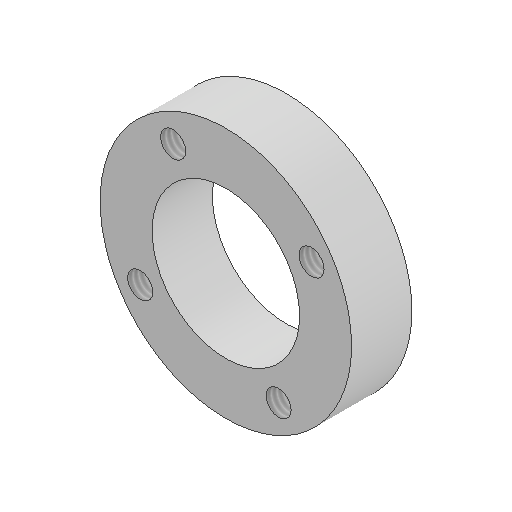
# Autodesk Inventor part: Part16
Saved by Autodesk Inventor 2024 (Build 280153000, 153)
## iProperties
Created: 2023-04-05
Part Number: Part16
Material: Generic
Document SubType Name: Modeling
Designer: ralph
Density: 1 g/cm^3
Appearance: Default
Author: ralph
Autodesk Inventor part; units mm, degrees
ref_plane "YZ Plane" through (0, 0, 0) normal (1, 0, 0) x (0, 1, 0)
ref_plane "XZ Plane" through (0, 0, 0) normal (0, 1, 0) x (-1, 0, 0)
ref_plane "XY Plane" through (0, 0, 0) normal (0, 0, 1) x (1, 0, 0)
sketch "Sketch1" plane through (0, 0, 0) normal (0, 0, 1) x (1, 0, 0)
  circle A0 centre (0, -5) radius 23.8125
  ellipse E0 centre (-25.0666, -29.0096) end of major axis (-17.3967, -26.4903) minor radius 5.8789 (-26.9076, -23.4263) -> (-26.9076, -23.4263) ccw projected
  line L0 (-26.9076, -23.4263) -> (-27.832, -23.7377) projected
  line L1 (-29.2659, -21.4083) -> (-28.5247, -20.677) projected
  ellipse E1 centre (-32.7272, -16.5643) end of major axis (-27.023, -10.8513) minor radius 5.8792 (-28.5715, -20.7232) -> (-28.5252, -20.6765) ccw projected
  ellipse E2 centre (-32.3466, -17.5895) end of major axis (-24.2964, -18.1971) minor radius 5.879 (-31.9108, -11.7266) -> (-31.9108, -11.7266) ccw projected
  line L2 (-31.9108, -11.7266) -> (-32.884, -11.6605) projected
  line L3 (-33.3173, -8.9597) -> (-32.3527, -8.5677) projected
  ellipse E3 centre (-34.6613, -3.1603) end of major axis (-27.2053, -0.0652) minor radius 5.8788 (-32.4136, -8.5925) -> (-32.353, -8.5671) ccw projected
  ellipse E4 centre (-34.7021, -4.2527) end of major axis (-41.907, -0.6107) minor radius 5.8791 (-32.0559, 0.9971) -> (-32.0559, 0.9971) ccw projected
  line L4 (-32.0559, 0.9971) -> (-32.9298, 1.4307) projected
  line L5 (-32.2965, 4.0917) -> (-31.2553, 4.0847) projected
  ellipse E5 centre (-31.3188, 9.9638) end of major axis (-23.246, 9.97) minor radius 5.8786 (-31.321, 4.0851) -> (-31.2553, 4.0853) ccw projected
  ellipse E6 centre (-31.7749, 8.9701) end of major axis (-37.0377, 15.0923) minor radius 5.8794 (-27.3208, 12.8079) -> (-27.3208, 12.8079) ccw projected
  line L6 (-27.3208, 12.8079) -> (-27.9622, 13.5428) projected
  line L7 (-26.3588, 15.759) -> (-25.3996, 15.3541) projected
  ellipse E7 centre (-23.2082, 20.8106) end of major axis (-30.6693, 23.8943) minor radius 5.8793 (-25.4601, 15.3796) -> (-25.3993, 15.3547) ccw projected
  ellipse E8 centre (-24.0096, 20.0665) end of major axis (-26.5289, 27.7364) minor radius 5.8789 (-18.4263, 21.9076) -> (-18.4263, 21.9076) ccw projected
  line L8 (-18.4263, 21.9076) -> (-18.7377, 22.832) projected
  line L9 (-16.4083, 24.2659) -> (-15.677, 23.5247) projected
  ellipse E9 centre (-11.5646, 27.7269) end of major axis (-17.2775, 33.4309) minor radius 5.8788 (-15.7232, 23.5715) -> (-15.6765, 23.5252) ccw projected
  ellipse E10 centre (-12.5894, 27.3465) end of major axis (-11.9818, 35.3967) minor radius 5.8789 (-6.7266, 26.9108) -> (-6.7266, 26.9108) ccw projected
  line L10 (-6.7266, 26.9108) -> (-6.6605, 27.884) projected
  line L11 (-3.9597, 28.3173) -> (-3.5677, 27.3527) projected
  ellipse E11 centre (1.8398, 29.6613) end of major axis (-1.2553, 37.1175) minor radius 5.879 (-3.5925, 27.4136) -> (-3.5671, 27.353) ccw projected
  ellipse E12 centre (0.7479, 29.7018) end of major axis (4.3898, 36.9062) minor radius 5.8783 (5.9971, 27.0559) -> (5.9971, 27.0559) ccw projected
  line L12 (5.9971, 27.0559) -> (6.4307, 27.9298) projected
  line L13 (9.0917, 27.2965) -> (9.0847, 26.2553) projected
  ellipse E13 centre (14.9639, 26.3188) end of major axis (14.9577, 34.3917) minor radius 5.8788 (9.0851, 26.321) -> (9.0853, 26.2553) ccw projected
  ellipse E14 centre (13.9703, 26.7747) end of major axis (20.0923, 32.0374) minor radius 5.8792 (17.8079, 22.3208) -> (17.8079, 22.3208) ccw projected
  line L14 (17.8079, 22.3208) -> (18.5428, 22.9622) projected
  line L15 (20.759, 21.3588) -> (20.3541, 20.3996) projected
  ellipse E15 centre (25.8103, 18.2083) end of major axis (28.8939, 25.6692) minor radius 5.879 (20.3796, 20.4601) -> (20.3547, 20.3993) ccw projected
  ellipse E16 centre (25.0664, 19.0099) end of major axis (32.7365, 21.5293) minor radius 5.8793 (26.9076, 13.4263) -> (26.9076, 13.4263) ccw projected
  line L16 (26.9076, 13.4263) -> (27.832, 13.7377) projected
  line L17 (29.2659, 11.4083) -> (28.5247, 10.677) projected
  ellipse E17 centre (32.7273, 6.5642) end of major axis (38.4316, 12.2773) minor radius 5.8794 (28.5715, 10.7232) -> (28.5252, 10.6765) ccw projected
  ellipse E18 centre (32.3466, 7.5897) end of major axis (40.3969, 6.9821) minor radius 5.8792 (31.9108, 1.7266) -> (31.9108, 1.7266) ccw projected
  line L18 (31.9108, 1.7266) -> (32.884, 1.6605) projected
  line L19 (33.3173, -1.0403) -> (32.3527, -1.4323) projected
  ellipse E19 centre (34.6614, -6.8401) end of major axis (42.1177, -3.7449) minor radius 5.8793 (32.4136, -1.4075) -> (32.353, -1.4329) ccw projected
  ellipse E20 centre (34.702, -5.7476) end of major axis (27.4973, -2.1056) minor radius 5.8787 (32.0559, -10.9971) -> (32.0559, -10.9971) ccw projected
  line L20 (32.0559, -10.9971) -> (32.9298, -11.4307) projected
  line L21 (32.2965, -14.0917) -> (31.2553, -14.0847) projected
  ellipse E21 centre (31.3188, -19.9647) end of major axis (39.3922, -19.9584) minor radius 5.8795 (31.321, -14.0851) -> (31.2553, -14.0853) ccw projected
  ellipse E22 centre (31.7746, -18.9703) end of major axis (26.5119, -12.8483) minor radius 5.8791 (27.3208, -22.8079) -> (27.3208, -22.8079) ccw projected
  line L22 (27.3208, -22.8079) -> (27.9622, -23.5428) projected
  line L23 (26.3588, -25.759) -> (25.3996, -25.3541) projected
  ellipse E23 centre (23.2082, -30.8104) end of major axis (15.7472, -27.7267) minor radius 5.8792 (25.4601, -25.3796) -> (25.3993, -25.3547) ccw projected
  ellipse E24 centre (24.0098, -30.0665) end of major axis (21.4905, -22.3965) minor radius 5.8792 (18.4263, -31.9076) -> (18.4263, -31.9076) ccw projected
  line L24 (18.4263, -31.9076) -> (18.7377, -32.832) projected
  line L25 (16.4083, -34.2659) -> (15.677, -33.5247) projected
  ellipse E25 centre (11.5644, -37.7271) end of major axis (5.8515, -32.0229) minor radius 5.8791 (15.7232, -33.5715) -> (15.6765, -33.5252) ccw projected
  ellipse E26 centre (12.5894, -37.3465) end of major axis (13.197, -29.2964) minor radius 5.879 (6.7266, -36.9108) -> (6.7266, -36.9108) ccw projected
  line L26 (6.7266, -36.9108) -> (6.6605, -37.884) projected
  line L27 (3.9597, -38.3173) -> (3.5677, -37.3527) projected
  ellipse E27 centre (-1.84, -39.6614) end of major axis (-4.9353, -32.2052) minor radius 5.8792 (3.5925, -37.4136) -> (3.5671, -37.353) ccw projected
  ellipse E28 centre (-0.7476, -39.702) end of major axis (2.8944, -32.4973) minor radius 5.8788 (-5.9971, -37.0559) -> (-5.9971, -37.0559) ccw projected
  line L28 (-5.9971, -37.0559) -> (-6.4307, -37.9298) projected
  line L29 (-9.0917, -37.2965) -> (-9.0847, -36.2553) projected
  ellipse E29 centre (-14.9646, -36.3188) end of major axis (-14.9708, -28.2455) minor radius 5.8794 (-9.0851, -36.321) -> (-9.0853, -36.2553) ccw projected
  ellipse E30 centre (-13.9704, -36.7745) end of major axis (-7.8485, -31.5119) minor radius 5.8789 (-17.8079, -32.3208) -> (-17.8079, -32.3208) ccw projected
  line L30 (-17.8079, -32.3208) -> (-18.5428, -32.9622) projected
  line L31 (-20.759, -31.3588) -> (-20.3541, -30.3996) projected
  ellipse E31 centre (-25.8105, -28.2082) end of major axis (-22.7268, -20.7472) minor radius 5.8792 (-20.3796, -30.4601) -> (-20.3547, -30.3993) ccw projected
  arc A1 (-20.3547, -30.3993) -> (-19.6444, -27.7629) centre (-30.6222, -26.2195) ccw projected
  arc A2 (-19.6444, -27.7629) -> (-24.163, -22.8941) centre (-23.8575, -27.1418) ccw projected
  arc A3 (-24.163, -22.8941) -> (-26.8451, -23.406) centre (-23.4417, -33.9564) ccw projected
  arc A4 (-28.5252, -20.6765) -> (-26.86, -18.5126) centre (-36.4116, -12.8856) ccw projected
  arc A5 (-26.86, -18.5126) -> (-29.1715, -12.2852) centre (-30.5148, -16.3265) ccw projected
  arc A6 (-29.1715, -12.2852) -> (-31.8453, -11.7317) centre (-32.7384, -22.7815) ccw projected
  arc A7 (-32.353, -8.5671) -> (-29.9865, -7.2051) centre (-36.6576, 1.6488) ccw projected
  arc A8 (-29.9865, -7.2051) -> (-29.7389, -0.5672) centre (-32.5264, -3.7868) ccw projected
  arc A9 (-29.7389, -0.5672) -> (-31.9973, 0.9673) centre (-37.0511, -8.8995) ccw projected
  arc A10 (-31.2553, 4.0853) -> (-28.5477, 4.4381) centre (-31.3228, 15.1709) ccw projected
  arc A11 (-28.5477, 4.4381) -> (-25.7788, 10.4759) centre (-29.5862, 8.5682) ccw projected
  arc A12 (-25.7788, 10.4759) -> (-27.2781, 12.758) centre (-35.723, 5.5762) ccw projected
  arc A13 (-25.3993, 15.3547) -> (-22.7629, 14.6444) centre (-21.2195, 25.6222) ccw projected
  arc A14 (-22.7629, 14.6444) -> (-17.8941, 19.163) centre (-22.1418, 18.8575) ccw projected
  arc A15 (-17.8941, 19.163) -> (-18.406, 21.8451) centre (-28.9564, 18.4417) ccw projected
  arc A16 (-15.6765, 23.5252) -> (-13.5126, 21.86) centre (-7.8856, 31.4116) ccw projected
  arc A17 (-13.5126, 21.86) -> (-7.2852, 24.1715) centre (-11.3265, 25.5148) ccw projected
  arc A18 (-7.2852, 24.1715) -> (-6.7317, 26.8453) centre (-17.7815, 27.7384) ccw projected
  arc A19 (-3.5671, 27.353) -> (-2.2051, 24.9865) centre (6.6488, 31.6576) ccw projected
  arc A20 (-2.2051, 24.9865) -> (4.4328, 24.7389) centre (1.2132, 27.5264) ccw projected
  arc A21 (4.4328, 24.7389) -> (5.9673, 26.9973) centre (-3.8995, 32.0511) ccw projected
  arc A22 (9.0853, 26.2553) -> (9.4381, 23.5477) centre (20.1709, 26.3228) ccw projected
  arc A23 (9.4381, 23.5477) -> (15.4759, 20.7788) centre (13.5682, 24.5862) ccw projected
  arc A24 (15.4759, 20.7788) -> (17.758, 22.2781) centre (10.5762, 30.723) ccw projected
  arc A25 (20.3547, 20.3993) -> (19.6444, 17.7629) centre (30.6222, 16.2195) ccw projected
  arc A26 (19.6444, 17.7629) -> (24.163, 12.8941) centre (23.8575, 17.1418) ccw projected
  arc A27 (24.163, 12.8941) -> (26.8451, 13.406) centre (23.4417, 23.9564) ccw projected
  arc A28 (28.5252, 10.6765) -> (26.86, 8.5126) centre (36.4116, 2.8856) ccw projected
  arc A29 (26.86, 8.5126) -> (29.1715, 2.2852) centre (30.5148, 6.3265) ccw projected
  arc A30 (29.1715, 2.2852) -> (31.8453, 1.7317) centre (32.7384, 12.7815) ccw projected
  arc A31 (32.353, -1.4329) -> (29.9865, -2.7949) centre (36.6576, -11.6488) ccw projected
  arc A32 (29.9865, -2.7949) -> (29.7389, -9.4328) centre (32.5264, -6.2132) ccw projected
  arc A33 (29.7389, -9.4328) -> (31.9973, -10.9673) centre (37.0511, -1.1005) ccw projected
  arc A34 (31.2553, -14.0853) -> (28.5477, -14.4381) centre (31.3228, -25.1709) ccw projected
  arc A35 (28.5477, -14.4381) -> (25.7788, -20.4759) centre (29.5862, -18.5682) ccw projected
  arc A36 (25.7788, -20.4759) -> (27.2781, -22.758) centre (35.723, -15.5762) ccw projected
  arc A37 (25.3993, -25.3547) -> (22.7629, -24.6444) centre (21.2195, -35.6222) ccw projected
  arc A38 (22.7629, -24.6444) -> (17.8941, -29.163) centre (22.1418, -28.8575) ccw projected
  arc A39 (17.8941, -29.163) -> (18.406, -31.8451) centre (28.9564, -28.4417) ccw projected
  arc A40 (15.6765, -33.5252) -> (13.5126, -31.86) centre (7.8856, -41.4116) ccw projected
  arc A41 (13.5126, -31.86) -> (7.2852, -34.1715) centre (11.3265, -35.5148) ccw projected
  arc A42 (7.2852, -34.1715) -> (6.7317, -36.8453) centre (17.7815, -37.7384) ccw projected
  arc A43 (3.5671, -37.353) -> (2.2051, -34.9865) centre (-6.6488, -41.6576) ccw projected
  arc A44 (2.2051, -34.9865) -> (-4.4328, -34.7389) centre (-1.2132, -37.5264) ccw projected
  arc A45 (-4.4328, -34.7389) -> (-5.9673, -36.9973) centre (3.8995, -42.0511) ccw projected
  arc A46 (-9.0853, -36.2553) -> (-9.4381, -33.5477) centre (-20.1709, -36.3228) ccw projected
  arc A47 (-9.4381, -33.5477) -> (-15.4759, -30.7788) centre (-13.5682, -34.5862) ccw projected
  arc A48 (-15.4759, -30.7788) -> (-17.758, -32.2781) centre (-10.5762, -40.723) ccw projected
  circle A49 centre (0, -5) radius 13.97 projected
  arc A50 (-30.4448, -24.1016) -> (-27.832, -23.7377) centre (-30.1027, -16.9958) ccw projected
  arc A51 (-30.7677, -23.577) -> (-30.4448, -24.1016) centre (0, -5) ccw projected
  arc A52 (-29.2659, -21.4083) -> (-30.7677, -23.577) centre (-24.2695, -26.4724) ccw projected
  arc A53 (-35.4372, -10.9969) -> (-32.884, -11.6605) centre (-32.4019, -4.5629) ccw projected
  arc A54 (-35.5347, -10.3886) -> (-35.4372, -10.9969) centre (0, -5) ccw projected
  arc A55 (-33.3173, -8.9597) -> (-35.5347, -10.3886) centre (-30.6393, -15.5504) ccw projected
  arc A56 (-35.0346, 3.0208) -> (-32.9298, 1.4307) centre (-29.7682, 7.8035) ccw projected
  arc A57 (-34.892, 3.6201) -> (-35.0346, 3.0208) centre (0, -5) ccw projected
  arc A58 (-32.2965, 4.0917) -> (-34.892, 3.6201) centre (-32.3444, -3.0221) ccw projected
  arc A59 (-29.2983, 15.8174) -> (-27.9622, 13.5428) centre (-22.6025, 18.2207) ccw projected
  arc A60 (-28.9372, 16.3165) -> (-29.2983, 15.8174) centre (0, -5) ccw projected
  arc A61 (-26.3588, 15.759) -> (-28.9372, 16.3165) centre (-29.1255, 9.205) ccw projected
  arc A62 (-19.1016, 25.4448) -> (-18.7377, 22.832) centre (-11.9958, 25.1027) ccw projected
  arc A63 (-18.577, 25.7677) -> (-19.1016, 25.4448) centre (0, -5) ccw projected
  arc A64 (-16.4083, 24.2659) -> (-18.577, 25.7677) centre (-21.4724, 19.2695) ccw projected
  arc A65 (-5.9969, 30.4372) -> (-6.6605, 27.884) centre (0.4371, 27.4019) ccw projected
  arc A66 (-5.3886, 30.5347) -> (-5.9969, 30.4372) centre (0, -5) ccw projected
  arc A67 (-3.9597, 28.3173) -> (-5.3886, 30.5347) centre (-10.5504, 25.6393) ccw projected
  arc A68 (8.0208, 30.0346) -> (6.4307, 27.9298) centre (12.8035, 24.7682) ccw projected
  arc A69 (8.6201, 29.892) -> (8.0208, 30.0346) centre (0, -5) ccw projected
  arc A70 (9.0917, 27.2965) -> (8.6201, 29.892) centre (1.9779, 27.3444) ccw projected
  arc A71 (20.8174, 24.2983) -> (18.5428, 22.9622) centre (23.2207, 17.6025) ccw projected
  arc A72 (21.3165, 23.9372) -> (20.8174, 24.2983) centre (0, -5) ccw projected
  arc A73 (20.759, 21.3588) -> (21.3165, 23.9372) centre (14.205, 24.1255) ccw projected
  arc A74 (30.4448, 14.1016) -> (27.832, 13.7377) centre (30.1027, 6.9958) ccw projected
  arc A75 (30.7677, 13.577) -> (30.4448, 14.1016) centre (0, -5) ccw projected
  arc A76 (29.2659, 11.4083) -> (30.7677, 13.577) centre (24.2695, 16.4724) ccw projected
  arc A77 (35.4372, 0.9969) -> (32.884, 1.6605) centre (32.4019, -5.4371) ccw projected
  arc A78 (35.5347, 0.3886) -> (35.4372, 0.9969) centre (0, -5) ccw projected
  arc A79 (33.3173, -1.0403) -> (35.5347, 0.3886) centre (30.6393, 5.5504) ccw projected
  arc A80 (35.0346, -13.0208) -> (32.9298, -11.4307) centre (29.7682, -17.8035) ccw projected
  arc A81 (34.892, -13.6201) -> (35.0346, -13.0208) centre (0, -5) ccw projected
  arc A82 (32.2965, -14.0917) -> (34.892, -13.6201) centre (32.3444, -6.9779) ccw projected
  arc A83 (29.2983, -25.8174) -> (27.9622, -23.5428) centre (22.6025, -28.2207) ccw projected
  arc A84 (28.9372, -26.3165) -> (29.2983, -25.8174) centre (0, -5) ccw projected
  arc A85 (26.3588, -25.759) -> (28.9372, -26.3165) centre (29.1255, -19.205) ccw projected
  arc A86 (19.1016, -35.4448) -> (18.7377, -32.832) centre (11.9958, -35.1027) ccw projected
  arc A87 (18.577, -35.7677) -> (19.1016, -35.4448) centre (0, -5) ccw projected
  arc A88 (16.4083, -34.2659) -> (18.577, -35.7677) centre (21.4724, -29.2695) ccw projected
  arc A89 (5.9969, -40.4372) -> (6.6605, -37.884) centre (-0.4371, -37.4019) ccw projected
  arc A90 (5.3886, -40.5347) -> (5.9969, -40.4372) centre (0, -5) ccw projected
  arc A91 (3.9597, -38.3173) -> (5.3886, -40.5347) centre (10.5504, -35.6393) ccw projected
  arc A92 (-8.0208, -40.0346) -> (-6.4307, -37.9298) centre (-12.8035, -34.7682) ccw projected
  arc A93 (-8.6201, -39.892) -> (-8.0208, -40.0346) centre (0, -5) ccw projected
  arc A94 (-9.0917, -37.2965) -> (-8.6201, -39.892) centre (-1.9779, -37.3444) ccw projected
  arc A95 (-20.8174, -34.2983) -> (-18.5428, -32.9622) centre (-23.2207, -27.6025) ccw projected
  arc A96 (-21.3165, -33.9372) -> (-20.8174, -34.2983) centre (0, -5) ccw projected
  arc A97 (-20.759, -31.3588) -> (-21.3165, -33.9372) centre (-14.205, -34.1255) ccw projected
  circle A98 centre (16.223, 4.9859) radius 2.3812 projected
  circle A99 centre (9.9859, -21.223) radius 2.3812 projected
  circle A100 centre (-9.9859, 11.223) radius 2.3812 projected
  circle A101 centre (-16.223, -14.9859) radius 2.3812 projected
  point P0 (0, 0)
  dimension "d0" = 47.625
  constraints: 1 centre point, 32 other
  measures "d0" diameter of A0
extrude "Extrusion1" add sketch "Sketch1" along normal blind 9.525 contours A0 | A49 | A98 | A99 | A100 | A101
sketch "Sketch2" plane through (0, -5, 9.525) normal (0, 0, 1) x (1, 0, 0)
  circle A0 centre (0, 0) radius 13.97
  point P0 (0, 5)
  dimension "d3" = 27.94
  constraints: 1 centre point
  measures "d3" diameter of A0
extrude "Extrusion2" cut sketch "Sketch2" against normal blind 26.9875
sketch "Sketch3" plane through (0, -5, 9.525) normal (0, 0, 1) x (1, 0, 0)
  circle A0 centre (0, 0) radius 13.97 projected
  circle A1 centre (0, 0) radius 23.8125 projected
  point P0 (0, 5)
extrude "Extrusion3" add sketch "Sketch3" against normal blind 11.43
sketch "Sketch4" plane through (0, -5, 9.525) normal (0, 0, 1) x (1, 0, 0)
  circle A0 centre (16.223, 9.9859) radius 2.3812 projected
  circle A1 centre (9.9859, -16.223) radius 2.3812 projected
  circle A2 centre (-9.9859, 16.223) radius 2.3812 projected
  circle A3 centre (-16.223, -9.9859) radius 2.3812 projected
  circle A4 centre (0, 0) radius 13.97 projected
  arc A5 (32.353, 3.5671) -> (31.8453, 6.7317) centre (0, 0) ccw projected
  arc A6 (29.1715, 7.2852) -> (31.8453, 6.7317) centre (32.7384, 17.7815) ccw projected
  arc A7 (26.86, 13.5126) -> (29.1715, 7.2852) centre (30.5148, 11.3265) ccw projected
  arc A8 (28.5252, 15.6765) -> (26.86, 13.5126) centre (36.4116, 7.8856) ccw projected
  arc A9 (28.5252, 15.6765) -> (26.8451, 18.406) centre (0, 0) ccw projected
  arc A10 (24.163, 17.8941) -> (26.8451, 18.406) centre (23.4417, 28.9564) ccw projected
  arc A11 (19.6444, 22.7629) -> (24.163, 17.8941) centre (23.8575, 22.1418) ccw projected
  arc A12 (20.3547, 25.3993) -> (19.6444, 22.7629) centre (30.6222, 21.2195) ccw projected
  arc A13 (20.3547, 25.3993) -> (17.758, 27.2781) centre (0, 0) ccw projected
  arc A14 (15.4759, 25.7788) -> (17.758, 27.2781) centre (10.5762, 35.723) ccw projected
  arc A15 (9.4381, 28.5477) -> (15.4759, 25.7788) centre (13.5682, 29.5862) ccw projected
  arc A16 (9.0853, 31.2553) -> (9.4381, 28.5477) centre (20.1709, 31.3228) ccw projected
  arc A17 (9.0853, 31.2553) -> (5.9673, 31.9973) centre (0, 0) ccw projected
  arc A18 (4.4328, 29.7389) -> (5.9673, 31.9973) centre (-3.8995, 37.0511) ccw projected
  arc A19 (-2.2051, 29.9865) -> (4.4328, 29.7389) centre (1.2132, 32.5264) ccw projected
  arc A20 (-3.5671, 32.353) -> (-2.2051, 29.9865) centre (6.6488, 36.6576) ccw projected
  arc A21 (-3.5671, 32.353) -> (-6.7317, 31.8453) centre (0, 0) ccw projected
  arc A22 (-7.2852, 29.1715) -> (-6.7317, 31.8453) centre (-17.7815, 32.7384) ccw projected
  arc A23 (-13.5126, 26.86) -> (-7.2852, 29.1715) centre (-11.3265, 30.5148) ccw projected
  arc A24 (-15.6765, 28.5252) -> (-13.5126, 26.86) centre (-7.8856, 36.4116) ccw projected
  arc A25 (-15.6765, 28.5252) -> (-18.406, 26.8451) centre (0, 0) ccw projected
  arc A26 (-17.8941, 24.163) -> (-18.406, 26.8451) centre (-28.9564, 23.4417) ccw projected
  arc A27 (-22.7629, 19.6444) -> (-17.8941, 24.163) centre (-22.1418, 23.8575) ccw projected
  arc A28 (-25.3993, 20.3547) -> (-22.7629, 19.6444) centre (-21.2195, 30.6222) ccw projected
  arc A29 (-25.3993, 20.3547) -> (-27.2781, 17.758) centre (0, 0) ccw projected
  arc A30 (-25.7788, 15.4759) -> (-27.2781, 17.758) centre (-35.723, 10.5762) ccw projected
  arc A31 (-28.5477, 9.4381) -> (-25.7788, 15.4759) centre (-29.5862, 13.5682) ccw projected
  arc A32 (-31.2553, 9.0853) -> (-28.5477, 9.4381) centre (-31.3228, 20.1709) ccw projected
  arc A33 (-31.2553, 9.0853) -> (-31.9973, 5.9673) centre (0, 0) ccw projected
  arc A34 (-29.7389, 4.4328) -> (-31.9973, 5.9673) centre (-37.0511, -3.8995) ccw projected
  arc A35 (-29.9865, -2.2051) -> (-29.7389, 4.4328) centre (-32.5264, 1.2132) ccw projected
  arc A36 (-32.353, -3.5671) -> (-29.9865, -2.2051) centre (-36.6576, 6.6488) ccw projected
  arc A37 (-32.353, -3.5671) -> (-31.8453, -6.7317) centre (0, 0) ccw projected
  arc A38 (-29.1715, -7.2852) -> (-31.8453, -6.7317) centre (-32.7384, -17.7815) ccw projected
  arc A39 (-26.86, -13.5126) -> (-29.1715, -7.2852) centre (-30.5148, -11.3265) ccw projected
  arc A40 (-28.5252, -15.6765) -> (-26.86, -13.5126) centre (-36.4116, -7.8856) ccw projected
  arc A41 (-28.5252, -15.6765) -> (-26.8451, -18.406) centre (0, 0) ccw projected
  arc A42 (-24.163, -17.8941) -> (-26.8451, -18.406) centre (-23.4417, -28.9564) ccw projected
  arc A43 (-19.6444, -22.7629) -> (-24.163, -17.8941) centre (-23.8575, -22.1418) ccw projected
  arc A44 (-20.3547, -25.3993) -> (-19.6444, -22.7629) centre (-30.6222, -21.2195) ccw projected
  arc A45 (-20.3547, -25.3993) -> (-17.758, -27.2781) centre (0, 0) ccw projected
  arc A46 (-15.4759, -25.7788) -> (-17.758, -27.2781) centre (-10.5762, -35.723) ccw projected
  arc A47 (-9.4381, -28.5477) -> (-15.4759, -25.7788) centre (-13.5682, -29.5862) ccw projected
  arc A48 (-9.0853, -31.2553) -> (-9.4381, -28.5477) centre (-20.1709, -31.3228) ccw projected
  arc A49 (-9.0853, -31.2553) -> (-5.9673, -31.9973) centre (0, 0) ccw projected
  arc A50 (-4.4328, -29.7389) -> (-5.9673, -31.9973) centre (3.8995, -37.0511) ccw projected
  arc A51 (2.2051, -29.9865) -> (-4.4328, -29.7389) centre (-1.2132, -32.5264) ccw projected
  arc A52 (3.5671, -32.353) -> (2.2051, -29.9865) centre (-6.6488, -36.6576) ccw projected
  arc A53 (3.5671, -32.353) -> (6.7317, -31.8453) centre (0, 0) ccw projected
  arc A54 (7.2852, -29.1715) -> (6.7317, -31.8453) centre (17.7815, -32.7384) ccw projected
  arc A55 (13.5126, -26.86) -> (7.2852, -29.1715) centre (11.3265, -30.5148) ccw projected
  arc A56 (15.6765, -28.5252) -> (13.5126, -26.86) centre (7.8856, -36.4116) ccw projected
  arc A57 (15.6765, -28.5252) -> (18.406, -26.8451) centre (0, 0) ccw projected
  arc A58 (17.8941, -24.163) -> (18.406, -26.8451) centre (28.9564, -23.4417) ccw projected
  arc A59 (22.7629, -19.6444) -> (17.8941, -24.163) centre (22.1418, -23.8575) ccw projected
  arc A60 (25.3993, -20.3547) -> (22.7629, -19.6444) centre (21.2195, -30.6222) ccw projected
  arc A61 (25.3993, -20.3547) -> (27.2781, -17.758) centre (0, 0) ccw projected
  arc A62 (25.7788, -15.4759) -> (27.2781, -17.758) centre (35.723, -10.5762) ccw projected
  arc A63 (28.5477, -9.4381) -> (25.7788, -15.4759) centre (29.5862, -13.5682) ccw projected
  arc A64 (31.2553, -9.0853) -> (28.5477, -9.4381) centre (31.3228, -20.1709) ccw projected
  arc A65 (31.2553, -9.0853) -> (31.9973, -5.9673) centre (0, 0) ccw projected
  arc A66 (29.7389, -4.4328) -> (31.9973, -5.9673) centre (37.0511, 3.8995) ccw projected
  arc A67 (29.9865, 2.2051) -> (29.7389, -4.4328) centre (32.5264, -1.2132) ccw projected
  arc A68 (32.353, 3.5671) -> (29.9865, 2.2051) centre (36.6576, -6.6488) ccw projected
  point P0 (0, 5)
extrude "Extrusion4" cut sketch "Sketch4" against normal blind 11.43 contours A0 | A1 | A2 | A3
thread "Thread1" size "10-24 UNC" class "2B" standard "ANSI Unified Screw Threads" full length
thread "Thread2" size "10-24 UNC" class "2B" standard "ANSI Unified Screw Threads" full length
thread "Thread3" size "10-24 UNC" class "2B" standard "ANSI Unified Screw Threads" full length
thread "Thread4" size "10-24 UNC" class "2B" standard "ANSI Unified Screw Threads" full length
body "Solid1"
